Autodesk Inventor part; units mm, degrees
(part 2 of 2)
sketch "Sketch8" plane through (0, 3, 0) normal (0, 1, 0) x (1, 0, 0)
  line L0 (-11.2204, -5.7631) -> (-11.2204, 54.2693) construction
  line L1 (-11.2204, 54.2693) -> (9.6224, 54.2693) construction
  line L2 (9.6224, 54.2693) -> (9.6224, -5.7631) construction
  line L3 (9.6224, -5.7631) -> (-11.2204, -5.7631) construction
  line L4 (6.2429, -26.0349) -> (6.2429, -5.5313) construction
  line L5 (6.2429, -5.5313) -> (7.2667, -5.5313) construction
  line L6 (7.2667, -5.5313) -> (7.2667, -26.0349) construction
  line L7 (7.2667, -26.0349) -> (6.2429, -26.0349) construction
  line L8 (-6.4941, -25.0536) -> (-6.4941, -13.8559) construction
  line L9 (-6.4941, -13.8559) -> (-2.7643, -13.8559) construction
  line L10 (-2.7643, -13.8559) -> (-2.7643, -25.0536) construction
  line L11 (-2.7643, -25.0536) -> (-6.4941, -25.0536) construction
  line L12 (12.3138, -0.177) -> (12.3138, 43.1958) construction
  line L13 (12.3138, 43.1958) -> (16.8916, 43.1958) construction
  line L14 (16.8916, 43.1958) -> (16.8916, -0.177) construction
  line L15 (16.8916, -0.177) -> (12.3138, -0.177) construction
  spline S0 degree 2 poles (-4.9481, 2.5804) (-1.7196, 2.5804) (1.3047, 0.7036) (1.3047, -1.251) knots 0 0 0 1 2 2 2
  spline S1 degree 2 poles (1.3047, -1.251) (1.3047, -3.2348) (-1.7779, -5.0922) (-4.9384, -5.0922) knots 0 0 0 1 2 2 2
  spline S2 degree 2 poles (-4.9384, -5.0922) (-8.1863, -5.0922) (-11.1912, -3.2153) (-11.1912, -1.251) knots 0 0 0 1 2 2 2
  spline S3 degree 2 poles (-11.1912, -1.251) (-11.1912, 0.7231) (-8.0794, 2.5804) (-4.9481, 2.5804) knots 0 0 0 1 2 2 2
  spline S4 degree 2 poles (-1.2917, 0.5189) (-1.8849, 0.7522) (-3.7131, 0.9467) (-4.9481, 0.9467) knots 0 0 0 1 2 2 2
  spline S5 degree 2 poles (-4.9481, 0.9467) (-6.1831, 0.9467) (-8.0016, 0.7522) (-8.6142, 0.5091) knots 0 0 0 1 2 2 2
  spline S6 degree 2 poles (-8.6142, 0.5091) (-9.2269, 0.266) (-9.859, -0.58) (-9.859, -1.251) knots 0 0 0 1 2 2 2
  spline S7 degree 2 poles (-9.859, -1.251) (-9.859, -1.922) (-9.2269, -2.7875) (-8.5948, -3.0403) knots 0 0 0 1 2 2 2
  spline S8 degree 2 poles (-8.5948, -3.0403) (-7.9821, -3.2834) (-6.115, -3.4584) (-4.9384, -3.4584) knots 0 0 0 1 2 2 2
  spline S9 degree 2 poles (-4.9384, -3.4584) (-3.6742, -3.4584) (-1.9821, -3.3029) (-1.3209, -3.05) knots 0 0 0 1 2 2 2
  spline S10 degree 2 poles (-1.3209, -3.05) (-0.6985, -2.8166) (-0.0275, -1.9512) (-0.0275, -1.251) knots 0 0 0 1 2 2 2
  spline S11 degree 2 poles (-0.0275, -1.251) (-0.0275, -0.5897) (-0.6596, 0.2757) (-1.2917, 0.5189) knots 0 0 0 1 2 2 2
  line L16 (1.0519, 6.6939) -> (1.0519, 4.7685)
  line L17 (1.0519, 4.7685) -> (-1.2431, 4.7685)
  line L18 (-1.2431, 4.7685) -> (-1.2431, 6.6939)
  line L19 (-1.2431, 6.6939) -> (1.0519, 6.6939)
  line L20 (-9.1491, 16.6518) -> (1.0519, 11.4589)
  line L21 (1.0519, 11.4589) -> (1.0519, 9.7474)
  line L22 (1.0519, 9.7474) -> (-9.538, 15.232)
  line L23 (-9.538, 15.232) -> (-9.538, 9.0375)
  line L24 (-9.538, 9.0375) -> (-10.9481, 9.0375)
  line L25 (-10.9481, 9.0375) -> (-10.9481, 16.6518)
  line L26 (-10.9481, 16.6518) -> (-9.1491, 16.6518)
  spline S12 degree 2 poles (1.3242, 21.7474) (1.3242, 20.8527) (0.7893, 19.3843) (0.2934, 18.8689) knots 0 0 0 1 2 2 2
  spline S13 degree 2 poles (0.2934, 18.8689) (-0.1928, 18.3633) (-1.5154, 17.8381) (-2.2641, 17.8381) knots 0 0 0 1 2 2 2
  spline S14 degree 2 poles (-2.2641, 17.8381) (-3.2366, 17.8381) (-4.8703, 18.8787) (-5.3565, 19.8706) knots 0 0 0 1 2 2 2
  line L27 (-5.3565, 19.8706) -> (-5.4051, 19.8706)
  spline S15 degree 2 poles (-5.4051, 19.8706) (-5.9205, 18.9856) (-7.1458, 18.1299) (-8.0599, 18.1299) knots 0 0 0 1 2 2 2
  spline S16 degree 2 poles (-8.0599, 18.1299) (-9.4116, 18.1299) (-11.2204, 20.172) (-11.2204, 21.7474) knots 0 0 0 1 2 2 2
  spline S17 degree 2 poles (-11.2204, 21.7474) (-11.2204, 23.3811) (-9.5089, 25.3552) (-8.1669, 25.3552) knots 0 0 0 1 2 2 2
  spline S18 degree 2 poles (-8.1669, 25.3552) (-7.3598, 25.3552) (-5.7844, 24.4119) (-5.3371, 23.527) knots 0 0 0 1 2 2 2
  line L28 (-5.3371, 23.527) -> (-5.2885, 23.527)
  spline S19 degree 2 poles (-5.2885, 23.527) (-4.8022, 24.5772) (-3.4019, 25.6566) (-2.2933, 25.6566) knots 0 0 0 1 2 2 2
  spline S20 degree 2 poles (-2.2933, 25.6566) (-0.7568, 25.6566) (1.3242, 23.42) (1.3242, 21.7474) knots 0 0 0 1 2 2 2
  spline S21 degree 2 poles (-2.1377, 24.0035) (-2.8768, 24.0035) (-3.752, 23.42) (-4.1993, 22.5934) knots 0 0 0 1 2 2 2
  spline S22 degree 2 poles (-4.1993, 22.5934) (-4.3549, 22.3211) (-4.7147, 21.407) (-4.9481, 20.8333) knots 0 0 0 1 2 2 2
  spline S23 degree 2 poles (-4.9481, 20.8333) (-4.5105, 20.172) (-3.2074, 19.4621) (-2.3808, 19.4621) knots 0 0 0 1 2 2 2
  spline S24 degree 2 poles (-2.3808, 19.4621) (-1.2917, 19.4621) (0.1281, 20.7749) (0.1281, 21.7668) knots 0 0 0 1 2 2 2
  spline S25 degree 2 poles (0.1281, 21.7668) (0.1281, 22.7782) (-1.0875, 24.0035) (-2.1377, 24.0035) knots 0 0 0 1 2 2 2
  spline S26 degree 2 poles (-8.1474, 23.7798) (-8.9546, 23.7798) (-10.034, 22.7004) (-10.034, 21.7377) knots 0 0 0 1 2 2 2
  spline S27 degree 2 poles (-10.034, 21.7377) (-10.034, 20.8625) (-9.0713, 19.7441) (-8.2447, 19.7441) knots 0 0 0 1 2 2 2
  spline S28 degree 2 poles (-8.2447, 19.7441) (-7.6515, 19.7441) (-6.8249, 20.3179) (-6.4943, 20.8916) knots 0 0 0 1 2 2 2
  spline S29 degree 2 poles (-6.4943, 20.8916) (-6.3581, 21.1347) (-5.8816, 22.1655) (-5.7455, 22.5837) knots 0 0 0 1 2 2 2
  spline S30 degree 2 poles (-5.7455, 22.5837) (-6.2803, 23.2839) (-7.4181, 23.7798) (-8.1474, 23.7798) knots 0 0 0 1 2 2 2
  line L29 (0.8179, -25.099) -> (-6.1821, -22.7392)
  line L30 (-6.1821, -22.7392) -> (-6.1821, -21.5933)
  line L31 (-6.1821, -21.5933) -> (0.8179, -19.2335)
  line L32 (0.8179, -19.2335) -> (0.8179, -20.2149)
  line L33 (0.8179, -20.2149) -> (-1.1391, -20.8502)
  line L34 (-1.1391, -20.8502) -> (-1.1391, -23.522)
  line L35 (-1.1391, -23.522) -> (0.8179, -24.1574)
  line L36 (0.8179, -24.1574) -> (0.8179, -25.099)
  line L37 (-1.9333, -21.1055) -> (-5.2291, -22.189)
  line L38 (-5.2291, -22.189) -> (-1.9333, -23.2668)
  line L39 (-1.9333, -23.2668) -> (-1.9333, -21.1055)
  spline S31 degree 2 poles (-1.8936, -14.236) (-0.6059, -14.236) (0.9654, -15.4839) (0.9654, -16.4256) knots 0 0 0 1 2 2 2
  spline S32 degree 2 poles (0.9654, -16.4256) (0.9654, -16.851) (0.7555, -17.458) (0.574, -17.753) knots 0 0 0 1 2 2 2
  line L40 (0.574, -17.753) -> (0.8179, -17.8097)
  line L41 (0.8179, -17.8097) -> (0.8179, -18.6379)
  line L42 (0.8179, -18.6379) -> (-6.4941, -18.6379)
  line L43 (-6.4941, -18.6379) -> (-6.4941, -17.753)
  line L44 (-6.4941, -17.753) -> (-3.8847, -17.753)
  spline S33 degree 2 poles (-3.8847, -17.753) (-4.1853, -17.4183) (-4.5824, -16.6411) (-4.5824, -16.1476) knots 0 0 0 1 2 2 2
  spline S34 degree 2 poles (-4.5824, -16.1476) (-4.5824, -15.257) (-3.1586, -14.236) (-1.8936, -14.236) knots 0 0 0 1 2 2 2
  spline S35 degree 2 poles (-1.8255, -15.1493) (-2.7672, -15.1493) (-3.7428, -15.7222) (-3.7428, -16.3575) knots 0 0 0 1 2 2 2
  spline S36 degree 2 poles (-3.7428, -16.3575) (-3.7428, -16.7149) (-3.4025, -17.4523) (-3.1415, -17.753) knots 0 0 0 1 2 2 2
  line L45 (-3.1415, -17.753) -> (-0.1294, -17.753)
  spline S37 degree 2 poles (-0.1294, -17.753) (0.0351, -17.4183) (0.1713, -16.9021) (0.1713, -16.5958) knots 0 0 0 1 2 2 2
  spline S38 degree 2 poles (0.1713, -16.5958) (0.1713, -15.9207) (-0.7874, -15.1493) (-1.8255, -15.1493) knots 0 0 0 1 2 2 2
  spline S39 degree 2 poles (0.9427, -11.8988) (0.9427, -12.4264) (0.6591, -13.3397) (0.5003, -13.6403) knots 0 0 0 1 2 2 2
  line L46 (0.5003, -13.6403) -> (-0.4924, -13.6403)
  line L47 (-0.4924, -13.6403) -> (-0.4924, -13.595)
  spline S40 degree 2 poles (-0.4924, -13.595) (-0.4017, -13.4815) (-0.1861, -13.1752) (-0.067, -12.9199) knots 0 0 0 1 2 2 2
  spline S41 degree 2 poles (-0.067, -12.9199) (0.0408, -12.6987) (0.1996, -12.1541) (0.1996, -11.8648) knots 0 0 0 1 2 2 2
  spline S42 degree 2 poles (0.1996, -11.8648) (0.1996, -11.6549) (0.1032, -11.1728) (0.0238, -11.0593) knots 0 0 0 1 2 2 2
  spline S43 degree 2 poles (0.0238, -11.0593) (-0.084, -10.8948) (-0.3279, -10.7473) (-0.5775, -10.7473) knots 0 0 0 1 2 2 2
  spline S44 degree 2 poles (-0.5775, -10.7473) (-0.8895, -10.7473) (-1.2129, -11.0877) (-1.3206, -11.5245) knots 0 0 0 1 2 2 2
  spline S45 degree 2 poles (-1.3206, -11.5245) (-1.3603, -11.6946) (-1.4738, -12.2392) (-1.5362, -12.4718) knots 0 0 0 1 2 2 2
  spline S46 degree 2 poles (-1.5362, -12.4718) (-1.712, -13.0731) (-2.4381, -13.6176) (-2.9543, -13.6176) knots 0 0 0 1 2 2 2
  spline S47 degree 2 poles (-2.9543, -13.6176) (-3.6691, -13.6176) (-4.5597, -12.5455) (-4.5597, -11.6606) knots 0 0 0 1 2 2 2
  spline S48 degree 2 poles (-4.5597, -11.6606) (-4.5597, -11.2238) (-4.3441, -10.3389) (-4.1796, -10.0382) knots 0 0 0 1 2 2 2
  line L48 (-4.1796, -10.0382) -> (-3.2323, -10.0382)
  line L49 (-3.2323, -10.0382) -> (-3.2323, -10.0836)
  spline S49 degree 2 poles (-3.2323, -10.0836) (-3.5046, -10.424) (-3.8166, -11.2522) (-3.8166, -11.6776) knots 0 0 0 1 2 2 2
  spline S50 degree 2 poles (-3.8166, -11.6776) (-3.8166, -12.1144) (-3.4479, -12.7157) (-3.0791, -12.7157) knots 0 0 0 1 2 2 2
  spline S51 degree 2 poles (-3.0791, -12.7157) (-2.7445, -12.7157) (-2.4211, -12.3583) (-2.319, -11.9612) knots 0 0 0 1 2 2 2
  spline S52 degree 2 poles (-2.319, -11.9612) (-2.268, -11.7684) (-2.1659, -11.2805) (-2.1035, -11.0139) knots 0 0 0 1 2 2 2
  spline S53 degree 2 poles (-2.1035, -11.0139) (-1.956, -10.4353) (-1.2809, -9.8454) (-0.6966, -9.8454) knots 0 0 0 1 2 2 2
  spline S54 degree 2 poles (-0.6966, -9.8454) (-0.3563, -9.8454) (0.245, -10.112) (0.4662, -10.3729) knots 0 0 0 1 2 2 2
  spline S55 degree 2 poles (0.4662, -10.3729) (0.6988, -10.6509) (0.9427, -11.3599) (0.9427, -11.8988) knots 0 0 0 1 2 2 2
  spline S56 degree 2 poles (9.9613, -24.3133) (9.9613, -24.6536) (9.7316, -25.2294) (9.5019, -25.4393) knots 0 0 0 1 2 2 2
  spline S57 degree 2 poles (9.5019, -25.4393) (9.275, -25.6492) (8.5942, -25.8789) (8.1518, -25.8789) knots 0 0 0 1 2 2 2
  spline S58 degree 2 poles (8.1518, -25.8789) (7.7122, -25.8789) (7.0598, -25.6548) (6.8187, -25.4421) knots 0 0 0 1 2 2 2
  spline S59 degree 2 poles (6.8187, -25.4421) (6.5833, -25.2322) (6.3365, -24.6593) (6.3365, -24.3048) knots 0 0 0 1 2 2 2
  spline S60 degree 2 poles (6.3365, -24.3048) (6.3365, -24.1289) (6.3876, -23.8197) (6.4273, -23.6893) knots 0 0 0 1 2 2 2
  spline S61 degree 2 poles (6.4273, -23.6893) (6.4642, -23.5758) (6.5691, -23.3404) (6.6315, -23.2241) knots 0 0 0 1 2 2 2
  line L50 (6.6315, -23.2241) -> (7.1931, -23.2241)
  line L51 (7.1931, -23.2241) -> (7.1931, -23.261)
  spline S62 degree 2 poles (7.1931, -23.261) (7.1364, -23.3234) (6.9775, -23.5163) (6.901, -23.6552) knots 0 0 0 1 2 2 2
  spline S63 degree 2 poles (6.901, -23.6552) (6.8272, -23.7885) (6.7336, -24.1034) (6.7336, -24.3076) knots 0 0 0 1 2 2 2
  spline S64 degree 2 poles (6.7336, -24.3076) (6.7336, -24.5317) (6.918, -24.9316) (7.0938, -25.0819) knots 0 0 0 1 2 2 2
  spline S65 degree 2 poles (7.0938, -25.0819) (7.2725, -25.2294) (7.8143, -25.3939) (8.1518, -25.3939) knots 0 0 0 1 2 2 2
  spline S66 degree 2 poles (8.1518, -25.3939) (8.512, -25.3939) (9.031, -25.2209) (9.2097, -25.0706) knots 0 0 0 1 2 2 2
  spline S67 degree 2 poles (9.2097, -25.0706) (9.3827, -24.9231) (9.5586, -24.5288) (9.5586, -24.3076) knots 0 0 0 1 2 2 2
  spline S68 degree 2 poles (9.5586, -24.3076) (9.5586, -24.1062) (9.4593, -23.763) (9.3856, -23.6297) knots 0 0 0 1 2 2 2
  spline S69 degree 2 poles (9.3856, -23.6297) (9.3118, -23.5021) (9.1587, -23.312) (9.1048, -23.2582) knots 0 0 0 1 2 2 2
  line L52 (9.1048, -23.2582) -> (9.1048, -23.2241)
  line L53 (9.1048, -23.2241) -> (9.6607, -23.2241)
  spline S70 degree 2 poles (9.6607, -23.2241) (9.7146, -23.3404) (9.8139, -23.5446) (9.8592, -23.6893) knots 0 0 0 1 2 2 2
  spline S71 degree 2 poles (9.8592, -23.6893) (9.9103, -23.8424) (9.9613, -24.1034) (9.9613, -24.3133) knots 0 0 0 1 2 2 2
  line L54 (9.8989, -20.7622) -> (9.8989, -21.2047)
  line L55 (9.8989, -21.2047) -> (8.4014, -21.2047)
  spline S72 degree 2 poles (8.4014, -21.2047) (8.2198, -21.2047) (7.9079, -21.2387) (7.8143, -21.2898) knots 0 0 0 1 2 2 2
  spline S73 degree 2 poles (7.8143, -21.2898) (7.715, -21.3437) (7.6186, -21.5365) (7.6186, -21.701) knots 0 0 0 1 2 2 2
  spline S74 degree 2 poles (7.6186, -21.701) (7.6186, -21.8655) (7.7944, -22.2144) (7.9362, -22.3817) knots 0 0 0 1 2 2 2
  line L56 (7.9362, -22.3817) -> (9.8989, -22.3817)
  line L57 (9.8989, -22.3817) -> (9.8989, -22.8242)
  line L58 (9.8989, -22.8242) -> (6.2429, -22.8242)
  line L59 (6.2429, -22.8242) -> (6.2429, -22.3817)
  line L60 (6.2429, -22.3817) -> (7.5647, -22.3817)
  spline S75 degree 2 poles (7.5647, -22.3817) (7.386, -22.1832) (7.1988, -21.8003) (7.1988, -21.5847) knots 0 0 0 1 2 2 2
  spline S76 degree 2 poles (7.1988, -21.5847) (7.1988, -21.199) (7.7093, -20.7622) (8.1943, -20.7622) knots 0 0 0 1 2 2 2
  line L61 (8.1943, -20.7622) -> (9.8989, -20.7622)
  spline S77 degree 2 poles (9.621, -18.6775) (9.6607, -18.7314) (9.8025, -18.9129) (9.8451, -18.998) knots 0 0 0 1 2 2 2
  spline S78 degree 2 poles (9.8451, -18.998) (9.9074, -19.1143) (9.9727, -19.3327) (9.9727, -19.5313) knots 0 0 0 1 2 2 2
  spline S79 degree 2 poles (9.9727, -19.5313) (9.9727, -19.6929) (9.8507, -19.9851) (9.7401, -20.0957) knots 0 0 0 1 2 2 2
  spline S80 degree 2 poles (9.7401, -20.0957) (9.6323, -20.2006) (9.3147, -20.3283) (9.1388, -20.3283) knots 0 0 0 1 2 2 2
  spline S81 degree 2 poles (9.1388, -20.3283) (8.8665, -20.3283) (8.4808, -20.0985) (8.3702, -19.8489) knots 0 0 0 1 2 2 2
  spline S82 degree 2 poles (8.3702, -19.8489) (8.2681, -19.6277) (8.1915, -19.0264) (8.1716, -18.6775) knots 0 0 0 1 2 2 2
  line L62 (8.1716, -18.6775) -> (8.0865, -18.6775)
  spline S83 degree 2 poles (8.0865, -18.6775) (7.9334, -18.6775) (7.7433, -18.7711) (7.6895, -18.8562) knots 0 0 0 1 2 2 2
  spline S84 degree 2 poles (7.6895, -18.8562) (7.6356, -18.9413) (7.6015, -19.1852) (7.6015, -19.3157) knots 0 0 0 1 2 2 2
  spline S85 degree 2 poles (7.6015, -19.3157) (7.6015, -19.4689) (7.6923, -19.883) (7.7802, -20.09) knots 0 0 0 1 2 2 2
  line L63 (7.7802, -20.09) -> (7.7802, -20.1155)
  line L64 (7.7802, -20.1155) -> (7.3292, -20.1155)
  spline S86 degree 2 poles (7.3292, -20.1155) (7.2952, -19.9936) (7.2101, -19.5369) (7.2101, -19.3129) knots 0 0 0 1 2 2 2
  spline S87 degree 2 poles (7.2101, -19.3129) (7.2101, -19.0406) (7.2952, -18.669) (7.4058, -18.5215) knots 0 0 0 1 2 2 2
  spline S88 degree 2 poles (7.4058, -18.5215) (7.5136, -18.3769) (7.8568, -18.2351) (8.1036, -18.2351) knots 0 0 0 1 2 2 2
  line L65 (8.1036, -18.2351) -> (9.8989, -18.2351)
  line L66 (9.8989, -18.2351) -> (9.8989, -18.6775)
  line L67 (9.8989, -18.6775) -> (9.621, -18.6775)
  line L68 (9.2523, -18.6775) -> (8.5233, -18.6775)
  spline S89 degree 2 poles (8.5233, -18.6775) (8.5375, -18.8364) (8.5857, -19.3157) (8.6311, -19.466) knots 0 0 0 1 2 2 2
  spline S90 degree 2 poles (8.6311, -19.466) (8.685, -19.6419) (8.9091, -19.8716) (9.1076, -19.8716) knots 0 0 0 1 2 2 2
  spline S91 degree 2 poles (9.1076, -19.8716) (9.3345, -19.8716) (9.5643, -19.6163) (9.5643, -19.3724) knots 0 0 0 1 2 2 2
  spline S92 degree 2 poles (9.5643, -19.3724) (9.5643, -19.1654) (9.3856, -18.825) (9.2523, -18.6775) knots 0 0 0 1 2 2 2
  line L69 (9.8989, -15.5519) -> (9.8989, -15.9944)
  line L70 (9.8989, -15.9944) -> (8.4014, -15.9944)
  spline S93 degree 2 poles (8.4014, -15.9944) (8.2198, -15.9944) (7.9079, -16.0284) (7.8143, -16.0795) knots 0 0 0 1 2 2 2
  spline S94 degree 2 poles (7.8143, -16.0795) (7.715, -16.1334) (7.6186, -16.3262) (7.6186, -16.4907) knots 0 0 0 1 2 2 2
  spline S95 degree 2 poles (7.6186, -16.4907) (7.6186, -16.6552) (7.7944, -17.0041) (7.9362, -17.1714) knots 0 0 0 1 2 2 2
  line L71 (7.9362, -17.1714) -> (9.8989, -17.1714)
  line L72 (9.8989, -17.1714) -> (9.8989, -17.6139)
  line L73 (9.8989, -17.6139) -> (7.2725, -17.6139)
  line L74 (7.2725, -17.6139) -> (7.2725, -17.1714)
  line L75 (7.2725, -17.1714) -> (7.5647, -17.1714)
  spline S96 degree 2 poles (7.5647, -17.1714) (7.386, -16.9729) (7.1988, -16.59) (7.1988, -16.3744) knots 0 0 0 1 2 2 2
  spline S97 degree 2 poles (7.1988, -16.3744) (7.1988, -15.9887) (7.7093, -15.5519) (8.1943, -15.5519) knots 0 0 0 1 2 2 2
  line L76 (8.1943, -15.5519) -> (9.8989, -15.5519)
  line L77 (9.8989, -12.8688) -> (9.8989, -13.3112)
  line L78 (9.8989, -13.3112) -> (8.4014, -13.3112)
  spline S98 degree 2 poles (8.4014, -13.3112) (8.2198, -13.3112) (7.9079, -13.3453) (7.8143, -13.3963) knots 0 0 0 1 2 2 2
  spline S99 degree 2 poles (7.8143, -13.3963) (7.715, -13.4502) (7.6186, -13.6431) (7.6186, -13.8076) knots 0 0 0 1 2 2 2
  spline S100 degree 2 poles (7.6186, -13.8076) (7.6186, -13.9721) (7.7944, -14.321) (7.9362, -14.4883) knots 0 0 0 1 2 2 2
  line L79 (7.9362, -14.4883) -> (9.8989, -14.4883)
  line L80 (9.8989, -14.4883) -> (9.8989, -14.9308)
  line L81 (9.8989, -14.9308) -> (7.2725, -14.9308)
  line L82 (7.2725, -14.9308) -> (7.2725, -14.4883)
  line L83 (7.2725, -14.4883) -> (7.5647, -14.4883)
  spline S101 degree 2 poles (7.5647, -14.4883) (7.386, -14.2898) (7.1988, -13.9069) (7.1988, -13.6913) knots 0 0 0 1 2 2 2
  spline S102 degree 2 poles (7.1988, -13.6913) (7.1988, -13.3056) (7.7093, -12.8688) (8.1943, -12.8688) knots 0 0 0 1 2 2 2
  line L84 (8.1943, -12.8688) -> (9.8989, -12.8688)
  spline S103 degree 2 poles (9.9585, -11.1074) (9.9585, -11.7371) (9.2523, -12.4291) (8.5999, -12.4291) knots 0 0 0 1 2 2 2
  spline S104 degree 2 poles (8.5999, -12.4291) (7.9589, -12.4291) (7.1988, -11.7569) (7.1988, -11.2152) knots 0 0 0 1 2 2 2
  spline S105 degree 2 poles (7.1988, -11.2152) (7.1988, -10.9713) (7.3406, -10.5941) (7.4909, -10.4551) knots 0 0 0 1 2 2 2
  spline S106 degree 2 poles (7.4909, -10.4551) (7.6412, -10.3133) (8.0752, -10.1629) (8.39, -10.1629) knots 0 0 0 1 2 2 2
  line L85 (8.39, -10.1629) -> (8.6311, -10.1629)
  line L86 (8.6311, -10.1629) -> (8.6311, -11.981)
  spline S107 degree 2 poles (8.6311, -11.981) (9.0878, -11.981) (9.5728, -11.5215) (9.5728, -11.1131) knots 0 0 0 1 2 2 2
  spline S108 degree 2 poles (9.5728, -11.1131) (9.5728, -10.9684) (9.5075, -10.6877) (9.4565, -10.5742) knots 0 0 0 1 2 2 2
  spline S109 degree 2 poles (9.4565, -10.5742) (9.3998, -10.4551) (9.3005, -10.2906) (9.2551, -10.2367) knots 0 0 0 1 2 2 2
  line L87 (9.2551, -10.2367) -> (9.2551, -10.2112)
  line L88 (9.2551, -10.2112) -> (9.7373, -10.2112)
  spline S110 degree 2 poles (9.7373, -10.2112) (9.7685, -10.2877) (9.8592, -10.5203) (9.8848, -10.6111) knots 0 0 0 1 2 2 2
  spline S111 degree 2 poles (9.8848, -10.6111) (9.9216, -10.7387) (9.9585, -10.9486) (9.9585, -11.1074) knots 0 0 0 1 2 2 2
  spline S112 degree 2 poles (8.2936, -10.5941) (8.1149, -10.5997) (7.854, -10.6735) (7.766, -10.7444) knots 0 0 0 1 2 2 2
  spline S113 degree 2 poles (7.766, -10.7444) (7.6668, -10.821) (7.5618, -11.062) (7.5618, -11.2407) knots 0 0 0 1 2 2 2
  spline S114 degree 2 poles (7.5618, -11.2407) (7.5618, -11.4166) (7.6668, -11.6633) (7.7689, -11.7655) knots 0 0 0 1 2 2 2
  spline S115 degree 2 poles (7.7689, -11.7655) (7.8738, -11.8647) (8.1263, -11.9668) (8.2936, -11.981) knots 0 0 0 1 2 2 2
  line L89 (8.2936, -11.981) -> (8.2936, -10.5941)
  line L90 (9.8989, -9.2638) -> (9.8989, -9.7063)
  line L91 (9.8989, -9.7063) -> (6.2429, -9.7063)
  line L92 (6.2429, -9.7063) -> (6.2429, -9.2638)
  line L93 (6.2429, -9.2638) -> (9.8989, -9.2638)
  line L94 (9.8989, -5.0179) -> (9.8989, -7.1763)
  line L95 (9.8989, -7.1763) -> (9.4026, -7.1763)
  spline S116 degree 2 poles (9.4026, -7.1763) (9.1842, -6.9437) (8.7786, -6.5296) (8.5602, -6.3311) knots 0 0 0 1 2 2 2
  spline S117 degree 2 poles (8.5602, -6.3311) (8.1206, -5.9312) (7.593, -5.639) (7.3122, -5.639) knots 0 0 0 1 2 2 2
  spline S118 degree 2 poles (7.3122, -5.639) (7.1647, -5.639) (6.9435, -5.7298) (6.8726, -5.812) knots 0 0 0 1 2 2 2
  spline S119 degree 2 poles (6.8726, -5.812) (6.8017, -5.8943) (6.7308, -6.1099) (6.7308, -6.2403) knots 0 0 0 1 2 2 2
  spline S120 degree 2 poles (6.7308, -6.2403) (6.7308, -6.3651) (6.7932, -6.6204) (6.8414, -6.7367) knots 0 0 0 1 2 2 2
  spline S121 degree 2 poles (6.8414, -6.7367) (6.8811, -6.836) (6.9946, -7.0203) (7.0343, -7.077) knots 0 0 0 1 2 2 2
  line L96 (7.0343, -7.077) -> (7.0343, -7.1026)
  line L97 (7.0343, -7.1026) -> (6.5351, -7.1026)
  spline S122 degree 2 poles (6.5351, -7.1026) (6.4642, -6.9579) (6.3252, -6.4389) (6.3252, -6.2063) knots 0 0 0 1 2 2 2
  spline S123 degree 2 poles (6.3252, -6.2063) (6.3252, -5.7156) (6.8442, -5.1625) (7.2867, -5.1625) knots 0 0 0 1 2 2 2
  spline S124 degree 2 poles (7.2867, -5.1625) (7.4938, -5.1625) (7.8398, -5.259) (7.9873, -5.3441) knots 0 0 0 1 2 2 2
  spline S125 degree 2 poles (7.9873, -5.3441) (8.1404, -5.4291) (8.4411, -5.6759) (8.5857, -5.812) knots 0 0 0 1 2 2 2
  spline S126 degree 2 poles (8.5857, -5.812) (8.8268, -6.0333) (9.343, -6.575) (9.4933, -6.7367) knots 0 0 0 1 2 2 2
  line L98 (9.4933, -6.7367) -> (9.4933, -5.0179)
  line L99 (9.4933, -5.0179) -> (9.8989, -5.0179)
  line L100 (15.6616, -23.6524) -> (15.6616, -24.1261)
  line L101 (15.6616, -24.1261) -> (13.7102, -24.821)
  line L102 (13.7102, -24.821) -> (15.6616, -25.5641)
  line L103 (15.6616, -25.5641) -> (15.6616, -26.0236)
  line L104 (15.6616, -26.0236) -> (13.1827, -25.0422)
  line L105 (13.1827, -25.0422) -> (12.0056, -25.5102)
  line L106 (12.0056, -25.5102) -> (12.0056, -25.0308)
  line L107 (12.0056, -25.0308) -> (15.6616, -23.6524)
  line L108 (14.8107, -20.5892) -> (14.8107, -23.1873)
  line L109 (14.8107, -23.1873) -> (14.4335, -23.1873)
  line L110 (14.4335, -23.1873) -> (14.4335, -20.5892)
  line L111 (14.4335, -20.5892) -> (14.8107, -20.5892)
  line L112 (13.8237, -20.5892) -> (13.8237, -23.1873)
  line L113 (13.8237, -23.1873) -> (13.4464, -23.1873)
  line L114 (13.4464, -23.1873) -> (13.4464, -20.5892)
  line L115 (13.4464, -20.5892) -> (13.8237, -20.5892)
  spline S127 degree 2 poles (14.5271, -17.6678) (14.7965, -17.6678) (15.2532, -17.8465) (15.4063, -17.9968) knots 0 0 0 1 2 2 2
  spline S128 degree 2 poles (15.4063, -17.9968) (15.568, -18.1528) (15.7353, -18.5442) (15.7353, -18.7796) knots 0 0 0 1 2 2 2
  spline S129 degree 2 poles (15.7353, -18.7796) (15.7353, -19.015) (15.5765, -19.4036) (15.4177, -19.5511) knots 0 0 0 1 2 2 2
  spline S130 degree 2 poles (15.4177, -19.5511) (15.2276, -19.7326) (14.5895, -19.9368) (14.1243, -19.9368) knots 0 0 0 1 2 2 2
  spline S131 degree 2 poles (14.1243, -19.9368) (13.6677, -19.9368) (12.9331, -19.7496) (12.6608, -19.5539) knots 0 0 0 1 2 2 2
  spline S132 degree 2 poles (12.6608, -19.5539) (12.3942, -19.3639) (12.0964, -18.7626) (12.0964, -18.3684) knots 0 0 0 1 2 2 2
  spline S133 degree 2 poles (12.0964, -18.3684) (12.0964, -18.2521) (12.1191, -18.0479) (12.1446, -17.9713) knots 0 0 0 1 2 2 2
  line L116 (12.1446, -17.9713) -> (12.5956, -17.9713)
  line L117 (12.5956, -17.9713) -> (12.5956, -17.9911)
  spline S134 degree 2 poles (12.5956, -17.9911) (12.5615, -18.0564) (12.502, -18.2946) (12.502, -18.4308) knots 0 0 0 1 2 2 2
  spline S135 degree 2 poles (12.502, -18.4308) (12.502, -18.8676) (13.0919, -19.4036) (13.6705, -19.4547) knots 0 0 0 1 2 2 2
  spline S136 degree 2 poles (13.6705, -19.4547) (13.5542, -19.2873) (13.4266, -18.9356) (13.4266, -18.7257) knots 0 0 0 1 2 2 2
  spline S137 degree 2 poles (13.4266, -18.7257) (13.4266, -18.5215) (13.5088, -18.2152) (13.6336, -18.0479) knots 0 0 0 1 2 2 2
  spline S138 degree 2 poles (13.6336, -18.0479) (13.7783, -17.855) (14.2264, -17.6678) (14.5271, -17.6678) knots 0 0 0 1 2 2 2
  spline S139 degree 2 poles (14.5469, -18.1443) (14.3314, -18.1443) (14.0392, -18.2578) (13.9371, -18.3826) knots 0 0 0 1 2 2 2
  spline S140 degree 2 poles (13.9371, -18.3826) (13.8634, -18.4761) (13.8152, -18.7087) (13.8152, -18.8307) knots 0 0 0 1 2 2 2
  spline S141 degree 2 poles (13.8152, -18.8307) (13.8152, -18.9952) (13.9144, -19.3043) (14.008, -19.4547) knots 0 0 0 1 2 2 2
  spline S142 degree 2 poles (14.008, -19.4547) (14.0591, -19.4575) (14.1555, -19.4632) (14.2293, -19.4632) knots 0 0 0 1 2 2 2
  spline S143 degree 2 poles (14.2293, -19.4632) (14.5923, -19.4632) (15.0376, -19.3214) (15.1539, -19.2136) knots 0 0 0 1 2 2 2
  spline S144 degree 2 poles (15.1539, -19.2136) (15.2645, -19.1143) (15.3524, -18.8988) (15.3524, -18.7768) knots 0 0 0 1 2 2 2
  spline S145 degree 2 poles (15.3524, -18.7768) (15.3524, -18.4932) (14.9497, -18.1443) (14.5469, -18.1443) knots 0 0 0 1 2 2 2
  spline S146 degree 2 poles (13.9116, -15.0754) (14.8533, -15.0754) (15.7353, -15.6228) (15.7353, -16.1929) knots 0 0 0 1 2 2 2
  spline S147 degree 2 poles (15.7353, -16.1929) (15.7353, -16.7715) (14.8362, -17.3133) (13.9144, -17.3133) knots 0 0 0 1 2 2 2
  spline S148 degree 2 poles (13.9144, -17.3133) (12.9671, -17.3133) (12.0907, -16.7659) (12.0907, -16.1929) knots 0 0 0 1 2 2 2
  spline S149 degree 2 poles (12.0907, -16.1929) (12.0907, -15.6172) (12.9983, -15.0754) (13.9116, -15.0754) knots 0 0 0 1 2 2 2
  spline S150 degree 2 poles (14.978, -15.6767) (14.805, -15.6086) (14.2718, -15.5519) (13.9116, -15.5519) knots 0 0 0 1 2 2 2
  spline S151 degree 2 poles (13.9116, -15.5519) (13.5514, -15.5519) (13.021, -15.6086) (12.8423, -15.6796) knots 0 0 0 1 2 2 2
  spline S152 degree 2 poles (12.8423, -15.6796) (12.6636, -15.7505) (12.4793, -15.9972) (12.4793, -16.1929) knots 0 0 0 1 2 2 2
  spline S153 degree 2 poles (12.4793, -16.1929) (12.4793, -16.3886) (12.6636, -16.6411) (12.848, -16.7148) knots 0 0 0 1 2 2 2
  spline S154 degree 2 poles (12.848, -16.7148) (13.0267, -16.7857) (13.5712, -16.8368) (13.9144, -16.8368) knots 0 0 0 1 2 2 2
  spline S155 degree 2 poles (13.9144, -16.8368) (14.2832, -16.8368) (14.7767, -16.7914) (14.9695, -16.7176) knots 0 0 0 1 2 2 2
  spline S156 degree 2 poles (14.9695, -16.7176) (15.1511, -16.6496) (15.3468, -16.3971) (15.3468, -16.1929) knots 0 0 0 1 2 2 2
  spline S157 degree 2 poles (15.3468, -16.1929) (15.3468, -16.0001) (15.1624, -15.7476) (14.978, -15.6767) knots 0 0 0 1 2 2 2
  spline S158 degree 2 poles (13.9116, -12.449) (14.8533, -12.449) (15.7353, -12.9964) (15.7353, -13.5665) knots 0 0 0 1 2 2 2
  spline S159 degree 2 poles (15.7353, -13.5665) (15.7353, -14.1451) (14.8362, -14.6868) (13.9144, -14.6868) knots 0 0 0 1 2 2 2
  spline S160 degree 2 poles (13.9144, -14.6868) (12.9671, -14.6868) (12.0907, -14.1394) (12.0907, -13.5665) knots 0 0 0 1 2 2 2
  spline S161 degree 2 poles (12.0907, -13.5665) (12.0907, -12.9907) (12.9983, -12.449) (13.9116, -12.449) knots 0 0 0 1 2 2 2
  spline S162 degree 2 poles (14.978, -13.0503) (14.805, -12.9822) (14.2718, -12.9255) (13.9116, -12.9255) knots 0 0 0 1 2 2 2
  spline S163 degree 2 poles (13.9116, -12.9255) (13.5514, -12.9255) (13.021, -12.9822) (12.8423, -13.0531) knots 0 0 0 1 2 2 2
  spline S164 degree 2 poles (12.8423, -13.0531) (12.6636, -13.124) (12.4793, -13.3708) (12.4793, -13.5665) knots 0 0 0 1 2 2 2
  spline S165 degree 2 poles (12.4793, -13.5665) (12.4793, -13.7622) (12.6636, -14.0146) (12.848, -14.0884) knots 0 0 0 1 2 2 2
  spline S166 degree 2 poles (12.848, -14.0884) (13.0267, -14.1593) (13.5712, -14.2103) (13.9144, -14.2103) knots 0 0 0 1 2 2 2
  spline S167 degree 2 poles (13.9144, -14.2103) (14.2832, -14.2103) (14.7767, -14.165) (14.9695, -14.0912) knots 0 0 0 1 2 2 2
  spline S168 degree 2 poles (14.9695, -14.0912) (15.1511, -14.0231) (15.3468, -13.7707) (15.3468, -13.5665) knots 0 0 0 1 2 2 2
  spline S169 degree 2 poles (15.3468, -13.5665) (15.3468, -13.3736) (15.1624, -13.1212) (14.978, -13.0503) knots 0 0 0 1 2 2 2
  line L118 (15.6616, -9.8736) -> (15.6616, -10.3161)
  line L119 (15.6616, -10.3161) -> (14.164, -10.3161)
  spline S170 degree 2 poles (14.164, -10.3161) (13.9825, -10.3161) (13.6705, -10.3501) (13.5769, -10.4012) knots 0 0 0 1 2 2 2
  spline S171 degree 2 poles (13.5769, -10.4012) (13.4776, -10.4551) (13.3812, -10.6479) (13.3812, -10.8125) knots 0 0 0 1 2 2 2
  spline S172 degree 2 poles (13.3812, -10.8125) (13.3812, -10.977) (13.5571, -11.3258) (13.6989, -11.4932) knots 0 0 0 1 2 2 2
  line L120 (13.6989, -11.4932) -> (15.6616, -11.4932)
  line L121 (15.6616, -11.4932) -> (15.6616, -11.9356)
  line L122 (15.6616, -11.9356) -> (13.0352, -11.9356)
  line L123 (13.0352, -11.9356) -> (13.0352, -11.4932)
  line L124 (13.0352, -11.4932) -> (13.3273, -11.4932)
  spline S173 degree 2 poles (13.3273, -11.4932) (13.1486, -11.2946) (12.9614, -10.9117) (12.9614, -10.6962) knots 0 0 0 1 2 2 2
  spline S174 degree 2 poles (12.9614, -10.6962) (12.9614, -10.3104) (13.472, -9.8736) (13.957, -9.8736) knots 0 0 0 1 2 2 2
  line L125 (13.957, -9.8736) -> (15.6616, -9.8736)
  line L126 (15.6616, -6.2744) -> (14.1413, -6.2744)
  spline S175 degree 2 poles (14.1413, -6.2744) (13.9598, -6.2744) (13.6507, -6.3027) (13.5656, -6.3481) knots 0 0 0 1 2 2 2
  spline S176 degree 2 poles (13.5656, -6.3481) (13.472, -6.3935) (13.3812, -6.5665) (13.3812, -6.7168) knots 0 0 0 1 2 2 2
  spline S177 degree 2 poles (13.3812, -6.7168) (13.3812, -6.853) (13.5486, -7.165) (13.7074, -7.3295) knots 0 0 0 1 2 2 2
  spline S178 degree 2 poles (13.7074, -7.3295) (13.7471, -7.3266) (13.8577, -7.321) (13.9315, -7.321) knots 0 0 0 1 2 2 2
  line L127 (13.9315, -7.321) -> (15.6616, -7.321)
  line L128 (15.6616, -7.321) -> (15.6616, -7.7634)
  line L129 (15.6616, -7.7634) -> (14.1413, -7.7634)
  spline S179 degree 2 poles (14.1413, -7.7634) (13.9598, -7.7634) (13.6507, -7.7918) (13.5656, -7.8372) knots 0 0 0 1 2 2 2
  spline S180 degree 2 poles (13.5656, -7.8372) (13.472, -7.8826) (13.3812, -8.0556) (13.3812, -8.2059) knots 0 0 0 1 2 2 2
  spline S181 degree 2 poles (13.3812, -8.2059) (13.3812, -8.3477) (13.5599, -8.6625) (13.6989, -8.81) knots 0 0 0 1 2 2 2
  line L130 (13.6989, -8.81) -> (15.6616, -8.81)
  line L131 (15.6616, -8.81) -> (15.6616, -9.2525)
  line L132 (15.6616, -9.2525) -> (13.0352, -9.2525)
  line L133 (13.0352, -9.2525) -> (13.0352, -8.81)
  line L134 (13.0352, -8.81) -> (13.3245, -8.81)
  spline S182 degree 2 poles (13.3245, -8.81) (13.1515, -8.637) (12.9614, -8.2967) (12.9614, -8.0924) knots 0 0 0 1 2 2 2
  spline S183 degree 2 poles (12.9614, -8.0924) (12.9614, -7.8599) (13.1742, -7.4996) (13.4152, -7.4061) knots 0 0 0 1 2 2 2
  spline S184 degree 2 poles (13.4152, -7.4061) (13.1912, -7.2047) (12.9614, -6.8246) (12.9614, -6.6034) knots 0 0 0 1 2 2 2
  spline S185 degree 2 poles (12.9614, -6.6034) (12.9614, -6.4332) (13.0664, -6.1552) (13.1855, -6.0531) knots 0 0 0 1 2 2 2
  spline S186 degree 2 poles (13.1855, -6.0531) (13.3046, -5.9482) (13.662, -5.8319) (13.9315, -5.8319) knots 0 0 0 1 2 2 2
  line L135 (13.9315, -5.8319) -> (15.6616, -5.8319)
  line L136 (15.6616, -5.8319) -> (15.6616, -6.2744)
  line L137 (16.8916, 1.4369) -> (16.8916, 0.2144)
  line L138 (16.8916, 0.2144) -> (12.3138, 0.2144)
  line L139 (12.3138, 0.2144) -> (12.3138, 1.4369)
  line L140 (12.3138, 1.4369) -> (12.6485, 1.4369)
  line L141 (12.6485, 1.4369) -> (12.6485, 0.6257)
  line L142 (12.6485, 0.6257) -> (16.557, 0.6257)
  line L143 (16.557, 0.6257) -> (16.557, 1.4369)
  line L144 (16.557, 1.4369) -> (16.8916, 1.4369)
  line L145 (13.8852, 4.0349) -> (14.1433, 3.8818)
  line L146 (14.1433, 3.8818) -> (13.6327, 3.1131)
  line L147 (13.6327, 3.1131) -> (14.4893, 3.1301)
  line L148 (14.4893, 3.1301) -> (14.4893, 2.8352)
  line L149 (14.4893, 2.8352) -> (13.6327, 2.8493)
  line L150 (13.6327, 2.8493) -> (14.1461, 2.0864)
  line L151 (14.1461, 2.0864) -> (13.888, 1.9304)
  line L152 (13.888, 1.9304) -> (13.4001, 2.7614)
  line L153 (13.4001, 2.7614) -> (12.9151, 1.9304)
  line L154 (12.9151, 1.9304) -> (12.657, 2.0864)
  line L155 (12.657, 2.0864) -> (13.1704, 2.8522)
  line L156 (13.1704, 2.8522) -> (12.3138, 2.8352)
  line L157 (12.3138, 2.8352) -> (12.3138, 3.1301)
  line L158 (12.3138, 3.1301) -> (13.1704, 3.1103)
  line L159 (13.1704, 3.1103) -> (12.6599, 3.8818)
  line L160 (12.6599, 3.8818) -> (12.918, 4.0349)
  line L161 (12.918, 4.0349) -> (13.4001, 3.2039)
  line L162 (13.4001, 3.2039) -> (13.8852, 4.0349)
  line L163 (16.8916, 5.7452) -> (16.8916, 4.5228)
  line L164 (16.8916, 4.5228) -> (16.557, 4.5228)
  line L165 (16.557, 4.5228) -> (16.557, 5.3339)
  line L166 (16.557, 5.3339) -> (12.6485, 5.3339)
  line L167 (12.6485, 5.3339) -> (12.6485, 4.5228)
  line L168 (12.6485, 4.5228) -> (12.3138, 4.5228)
  line L169 (12.3138, 4.5228) -> (12.3138, 5.7452)
  line L170 (12.3138, 5.7452) -> (16.8916, 5.7452)
  line L171 (16.8916, 12.2602) -> (16.8916, 11.0377)
  line L172 (16.8916, 11.0377) -> (12.3138, 11.0377)
  line L173 (12.3138, 11.0377) -> (12.3138, 12.2602)
  line L174 (12.3138, 12.2602) -> (12.6485, 12.2602)
  line L175 (12.6485, 12.2602) -> (12.6485, 11.449)
  line L176 (12.6485, 11.449) -> (16.557, 11.449)
  line L177 (16.557, 11.449) -> (16.557, 12.2602)
  line L178 (16.557, 12.2602) -> (16.8916, 12.2602)
  line L179 (13.8852, 14.8582) -> (14.1433, 14.7051)
  line L180 (14.1433, 14.7051) -> (13.6327, 13.9365)
  line L181 (13.6327, 13.9365) -> (14.4893, 13.9535)
  line L182 (14.4893, 13.9535) -> (14.4893, 13.6585)
  line L183 (14.4893, 13.6585) -> (13.6327, 13.6727)
  line L184 (13.6327, 13.6727) -> (14.1461, 12.9097)
  line L185 (14.1461, 12.9097) -> (13.888, 12.7537)
  line L186 (13.888, 12.7537) -> (13.4001, 13.5847)
  line L187 (13.4001, 13.5847) -> (12.9151, 12.7537)
  line L188 (12.9151, 12.7537) -> (12.657, 12.9097)
  line L189 (12.657, 12.9097) -> (13.1704, 13.6755)
  line L190 (13.1704, 13.6755) -> (12.3138, 13.6585)
  line L191 (12.3138, 13.6585) -> (12.3138, 13.9535)
  line L192 (12.3138, 13.9535) -> (13.1704, 13.9336)
  line L193 (13.1704, 13.9336) -> (12.6599, 14.7051)
  line L194 (12.6599, 14.7051) -> (12.918, 14.8582)
  line L195 (12.918, 14.8582) -> (13.4001, 14.0272)
  line L196 (13.4001, 14.0272) -> (13.8852, 14.8582)
  line L197 (16.8916, 16.5685) -> (16.8916, 15.3461)
  line L198 (16.8916, 15.3461) -> (16.557, 15.3461)
  line L199 (16.557, 15.3461) -> (16.557, 16.1573)
  line L200 (16.557, 16.1573) -> (12.6485, 16.1573)
  line L201 (12.6485, 16.1573) -> (12.6485, 15.3461)
  line L202 (12.6485, 15.3461) -> (12.3138, 15.3461)
  line L203 (12.3138, 15.3461) -> (12.3138, 16.5685)
  line L204 (12.3138, 16.5685) -> (16.8916, 16.5685)
  line L205 (16.8916, 24.5868) -> (16.8916, 23.3643)
  line L206 (16.8916, 23.3643) -> (12.3138, 23.3643)
  line L207 (12.3138, 23.3643) -> (12.3138, 24.5868)
  line L208 (12.3138, 24.5868) -> (12.6485, 24.5868)
  line L209 (12.6485, 24.5868) -> (12.6485, 23.7756)
  line L210 (12.6485, 23.7756) -> (16.557, 23.7756)
  line L211 (16.557, 23.7756) -> (16.557, 24.5868)
  line L212 (16.557, 24.5868) -> (16.8916, 24.5868)
  line L213 (16.8916, 29.2752) -> (16.8916, 28.0527)
  line L214 (16.8916, 28.0527) -> (16.557, 28.0527)
  line L215 (16.557, 28.0527) -> (16.557, 28.8639)
  line L216 (16.557, 28.8639) -> (12.6485, 28.8639)
  line L217 (12.6485, 28.8639) -> (12.6485, 28.0527)
  line L218 (12.6485, 28.0527) -> (12.3138, 28.0527)
  line L219 (12.3138, 28.0527) -> (12.3138, 29.2752)
  line L220 (12.3138, 29.2752) -> (16.8916, 29.2752)
  point P0 (0, 0)
  constraints: 8 other
emboss "Emboss1" sketch "Sketch8" operation add depth 0.1 direction (0, -1, 0)
body "Solid1"
